Autodesk Fusion 360 part; units mm, degrees
(part 3 of 3)
sketch "Sketch33" plane through (0, 0, 2.9845) normal (0, 0, 1) x (1, 0, 0)
  line L0 (32.131, 76.2) -> (38.1, 76.2)
  line L1 (38.1, 76.2) -> (38.1, 95.631)
  line L2 (38.1, 95.631) -> (32.131, 95.631)
  line L3 (32.131, 95.631) -> (32.131, 101.6)
  line L4 (32.131, 101.6) -> (38.1, 101.6)
  line L5 (38.1, 101.6) -> (38.1, 121.031)
  line L6 (38.1, 121.031) -> (32.131, 121.031)
  line L7 (32.131, 121.031) -> (32.131, 127)
  line L8 (32.131, 127) -> (38.1, 127)
  line L9 (38.1, 127) -> (38.1, 146.431)
  line L10 (38.1, 146.431) -> (32.131, 146.431)
  line L11 (32.131, 146.431) -> (32.131, 152.4)
  line L12 (32.131, 152.4) -> (38.1, 152.4)
  line L13 (38.1, 152.4) -> (38.1, 171.831)
  line L14 (38.1, 171.831) -> (32.131, 171.831)
  line L15 (32.131, 171.831) -> (32.131, 177.8)
  line L16 (32.131, 177.8) -> (38.1, 177.8)
  line L17 (38.1, 177.8) -> (38.1, 197.231)
  line L18 (38.1, 197.231) -> (32.131, 197.231)
  line L19 (32.131, 197.231) -> (32.131, 203.2)
  line L20 (32.131, 203.2) -> (38.1, 203.2)
  line L21 (38.1, 203.2) -> (38.1, 222.631)
  line L22 (38.1, 222.631) -> (32.131, 222.631)
  line L23 (32.131, 222.631) -> (32.131, 228.6)
  line L24 (32.131, 228.6) -> (38.1, 228.6)
  line L25 (38.1, 228.6) -> (38.1, 254)
  line L26 (38.1, 254) -> (31.75, 254)
  line L27 (31.75, 254) -> (31.75, 292.1)
  arc A0 (31.75, 292.1) -> (19.05, 304.8) centre (19.05, 292.1) ccw
  line L28 (19.05, 304.8) -> (-19.05, 304.8)
  arc A1 (-19.05, 304.8) -> (-31.75, 292.1) centre (-19.05, 292.1) ccw
  line L29 (-31.75, 292.1) -> (-31.75, 254)
  line L30 (-31.75, 254) -> (-38.1, 254)
  line L31 (-38.1, 254) -> (-38.1, 228.6)
  line L32 (-38.1, 228.6) -> (-32.131, 228.6)
  line L33 (-32.131, 228.6) -> (-32.131, 222.631)
  line L34 (-32.131, 222.631) -> (-38.1, 222.631)
  line L35 (-38.1, 222.631) -> (-38.1, 203.2)
  line L36 (-38.1, 203.2) -> (-32.131, 203.2)
  line L37 (-32.131, 203.2) -> (-32.131, 197.231)
  line L38 (-32.131, 197.231) -> (-38.1, 197.231)
  line L39 (-38.1, 197.231) -> (-38.1, 177.8)
  line L40 (-38.1, 177.8) -> (-32.131, 177.8)
  line L41 (-32.131, 177.8) -> (-32.131, 171.831)
  line L42 (-32.131, 171.831) -> (-38.1, 171.831)
  line L43 (-38.1, 171.831) -> (-38.1, 152.4)
  line L44 (-38.1, 152.4) -> (-32.131, 152.4)
  line L45 (-32.131, 152.4) -> (-32.131, 146.431)
  line L46 (-32.131, 146.431) -> (-38.1, 146.431)
  line L47 (-38.1, 146.431) -> (-38.1, 127)
  line L48 (-38.1, 127) -> (-32.131, 127)
  line L49 (-32.131, 127) -> (-32.131, 121.031)
  line L50 (-32.131, 121.031) -> (-38.1, 121.031)
  line L51 (-38.1, 121.031) -> (-38.1, 101.6)
  line L52 (-38.1, 101.6) -> (-32.131, 101.6)
  line L53 (-32.131, 101.6) -> (-32.131, 95.631)
  line L54 (-32.131, 95.631) -> (-38.1, 95.631)
  line L55 (-38.1, 95.631) -> (-38.1, 76.2)
  line L56 (-38.1, 76.2) -> (-32.131, 76.2)
  line L57 (-32.131, 76.2) -> (-32.131, 70.231)
  line L58 (-32.131, 70.231) -> (-38.1, 70.231)
  line L59 (-38.1, 70.231) -> (-38.1, 50.8)
  line L60 (-38.1, 50.8) -> (-32.131, 50.8)
  line L61 (-32.131, 50.8) -> (-32.131, 44.831)
  line L62 (-32.131, 44.831) -> (-38.1, 44.831)
  line L63 (-38.1, 44.831) -> (-38.1, 0)
  line L64 (-38.1, 0) -> (-88.9, 0)
  line L65 (-88.9, 0) -> (-88.9, 5.969)
  line L66 (-88.9, 5.969) -> (-114.3, 5.969)
  line L67 (-114.3, 5.969) -> (-114.3, -6.35)
  arc A2 (-114.3, -6.35) -> (-101.6, -19.05) centre (-101.6, -6.35) ccw
  line L68 (-101.6, -19.05) -> (-2.9845, -19.05)
  line L69 (-2.9845, -19.05) -> (-2.9845, -9.525)
  line L70 (-2.9845, -9.525) -> (2.9845, -9.525)
  line L71 (2.9845, -9.525) -> (2.9845, -19.05)
  line L72 (2.9845, -19.05) -> (101.6, -19.05)
  arc A3 (101.6, -19.05) -> (114.3, -6.35) centre (101.6, -6.35) ccw
  line L73 (114.3, -6.35) -> (114.3, 5.969)
  line L74 (114.3, 5.969) -> (88.9, 5.969)
  line L75 (88.9, 5.969) -> (88.9, 0)
  line L76 (88.9, 0) -> (38.1, 0)
  line L77 (38.1, 0) -> (38.1, 44.831)
  line L78 (38.1, 44.831) -> (32.131, 44.831)
  line L79 (32.131, 44.831) -> (32.131, 50.8)
  line L80 (32.131, 50.8) -> (38.1, 50.8)
  line L81 (38.1, 50.8) -> (38.1, 70.231)
  line L82 (38.1, 70.231) -> (32.131, 70.231)
  line L83 (32.131, 70.231) -> (32.131, 76.2)
  circle A4 centre (17.3609, 285.75) radius 11.1125
  circle A5 centre (-17.3609, 285.75) radius 11.1125
sketch "Sketch34" plane through (2.9845, 0, 0) normal (1, 0, 0) x (0, 0, -1)
  circle A0 centre (-17.3736, 285.75) radius 11.1125
  circle A1 centre (17.3736, 285.75) radius 11.1125
  line L0 (-38.1, 76.2) -> (-32.131, 76.2)
  line L1 (-32.131, 76.2) -> (-32.131, 70.231)
  line L2 (-32.131, 70.231) -> (-38.1, 70.231)
  line L3 (-38.1, 70.231) -> (-38.1, 50.8)
  line L4 (-38.1, 50.8) -> (-32.131, 50.8)
  line L5 (-32.131, 50.8) -> (-32.131, 44.831)
  line L6 (-32.131, 44.831) -> (-38.1, 44.831)
  line L7 (-38.1, 44.831) -> (-38.1, 0)
  line L8 (-38.1, 0) -> (-88.9, 0)
  line L9 (-88.9, 0) -> (-88.9, 5.969)
  line L10 (-88.9, 5.969) -> (-114.3, 5.969)
  line L11 (-114.3, 5.969) -> (-114.3, -6.35)
  arc A2 (-114.3, -6.35) -> (-101.6, -19.05) centre (-101.6, -6.35) ccw
  line L12 (-101.6, -19.05) -> (101.6, -19.05)
  arc A3 (101.6, -19.05) -> (114.3, -6.35) centre (101.6, -6.35) ccw
  line L13 (114.3, -6.35) -> (114.3, 5.969)
  line L14 (114.3, 5.969) -> (88.9, 5.969)
  line L15 (88.9, 5.969) -> (88.9, 0)
  line L16 (88.9, 0) -> (38.1, 0)
  line L17 (38.1, 0) -> (38.1, 44.831)
  line L18 (38.1, 44.831) -> (32.131, 44.831)
  line L19 (32.131, 44.831) -> (32.131, 50.8)
  line L20 (32.131, 50.8) -> (38.1, 50.8)
  line L21 (38.1, 50.8) -> (38.1, 70.231)
  line L22 (38.1, 70.231) -> (32.131, 70.231)
  line L23 (32.131, 70.231) -> (32.131, 76.2)
  line L24 (32.131, 76.2) -> (38.1, 76.2)
  line L25 (38.1, 76.2) -> (38.1, 95.631)
  line L26 (38.1, 95.631) -> (32.131, 95.631)
  line L27 (32.131, 95.631) -> (32.131, 101.6)
  line L28 (32.131, 101.6) -> (38.1, 101.6)
  line L29 (38.1, 101.6) -> (38.1, 121.031)
  line L30 (38.1, 121.031) -> (32.131, 121.031)
  line L31 (32.131, 121.031) -> (32.131, 127)
  line L32 (32.131, 127) -> (38.1, 127)
  line L33 (38.1, 127) -> (38.1, 146.431)
  line L34 (38.1, 146.431) -> (32.131, 146.431)
  line L35 (32.131, 146.431) -> (32.131, 152.4)
  line L36 (32.131, 152.4) -> (38.1, 152.4)
  line L37 (38.1, 152.4) -> (38.1, 171.831)
  line L38 (38.1, 171.831) -> (32.131, 171.831)
  line L39 (32.131, 171.831) -> (32.131, 177.8)
  line L40 (32.131, 177.8) -> (38.1, 177.8)
  line L41 (38.1, 177.8) -> (38.1, 197.231)
  line L42 (38.1, 197.231) -> (32.131, 197.231)
  line L43 (32.131, 197.231) -> (32.131, 203.2)
  line L44 (32.131, 203.2) -> (38.1, 203.2)
  line L45 (38.1, 203.2) -> (38.1, 222.631)
  line L46 (38.1, 222.631) -> (32.131, 222.631)
  line L47 (32.131, 222.631) -> (32.131, 228.6)
  line L48 (32.131, 228.6) -> (38.1, 228.6)
  line L49 (38.1, 228.6) -> (38.1, 254)
  line L50 (38.1, 254) -> (31.75, 254)
  line L51 (31.75, 254) -> (31.75, 292.1)
  arc A4 (31.75, 292.1) -> (19.05, 304.8) centre (19.05, 292.1) ccw
  line L52 (19.05, 304.8) -> (2.9845, 304.8)
  line L53 (2.9845, 304.8) -> (2.9845, -9.525)
  line L54 (2.9845, -9.525) -> (-2.9845, -9.525)
  line L55 (-2.9845, -9.525) -> (-2.9845, 304.8)
  line L56 (-2.9845, 304.8) -> (-19.05, 304.8)
  arc A5 (-19.05, 304.8) -> (-31.75, 292.1) centre (-19.05, 292.1) ccw
  line L57 (-31.75, 292.1) -> (-31.75, 254)
  line L58 (-31.75, 254) -> (-38.1, 254)
  line L59 (-38.1, 254) -> (-38.1, 228.6)
  line L60 (-38.1, 228.6) -> (-32.131, 228.6)
  line L61 (-32.131, 228.6) -> (-32.131, 222.631)
  line L62 (-32.131, 222.631) -> (-38.1, 222.631)
  line L63 (-38.1, 222.631) -> (-38.1, 203.2)
  line L64 (-38.1, 203.2) -> (-32.131, 203.2)
  line L65 (-32.131, 203.2) -> (-32.131, 197.231)
  line L66 (-32.131, 197.231) -> (-38.1, 197.231)
  line L67 (-38.1, 197.231) -> (-38.1, 177.8)
  line L68 (-38.1, 177.8) -> (-32.131, 177.8)
  line L69 (-32.131, 177.8) -> (-32.131, 171.831)
  line L70 (-32.131, 171.831) -> (-38.1, 171.831)
  line L71 (-38.1, 171.831) -> (-38.1, 152.4)
  line L72 (-38.1, 152.4) -> (-32.131, 152.4)
  line L73 (-32.131, 152.4) -> (-32.131, 146.431)
  line L74 (-32.131, 146.431) -> (-38.1, 146.431)
  line L75 (-38.1, 146.431) -> (-38.1, 127)
  line L76 (-38.1, 127) -> (-32.131, 127)
  line L77 (-32.131, 127) -> (-32.131, 121.031)
  line L78 (-32.131, 121.031) -> (-38.1, 121.031)
  line L79 (-38.1, 121.031) -> (-38.1, 101.6)
  line L80 (-38.1, 101.6) -> (-32.131, 101.6)
  line L81 (-32.131, 101.6) -> (-32.131, 95.631)
  line L82 (-32.131, 95.631) -> (-38.1, 95.631)
  line L83 (-38.1, 95.631) -> (-38.1, 76.2)
move_face "OffsetFaces2" offset -152.4 1 faces at (-0.9948, -9.525, 0.9948) on bodies 3 in component "Component'"
sketch "Sketch35" plane through (2.9845, 0, 0) normal (1, 0, 0) x (0, 0, -1)
  circle A0 centre (-17.3736, 285.75) radius 11.1125
  circle A1 centre (17.3736, 285.75) radius 11.1125
  line L0 (-38.1, 76.2) -> (-32.131, 76.2)
  line L1 (-32.131, 76.2) -> (-32.131, 70.231)
  line L2 (-32.131, 70.231) -> (-38.1, 70.231)
  line L3 (-38.1, 70.231) -> (-38.1, 50.8)
  line L4 (-38.1, 50.8) -> (-32.131, 50.8)
  line L5 (-32.131, 50.8) -> (-32.131, 44.831)
  line L6 (-32.131, 44.831) -> (-38.1, 44.831)
  line L7 (-38.1, 44.831) -> (-38.1, 0)
  line L8 (-38.1, 0) -> (-88.9, 0)
  line L9 (-88.9, 0) -> (-88.9, 5.969)
  line L10 (-88.9, 5.969) -> (-114.3, 5.969)
  line L11 (-114.3, 5.969) -> (-114.3, -6.35)
  arc A2 (-114.3, -6.35) -> (-101.6, -19.05) centre (-101.6, -6.35) ccw
  line L12 (-101.6, -19.05) -> (101.6, -19.05)
  arc A3 (101.6, -19.05) -> (114.3, -6.35) centre (101.6, -6.35) ccw
  line L13 (114.3, -6.35) -> (114.3, 5.969)
  line L14 (114.3, 5.969) -> (88.9, 5.969)
  line L15 (88.9, 5.969) -> (88.9, 0)
  line L16 (88.9, 0) -> (38.1, 0)
  line L17 (38.1, 0) -> (38.1, 44.831)
  line L18 (38.1, 44.831) -> (32.131, 44.831)
  line L19 (32.131, 44.831) -> (32.131, 50.8)
  line L20 (32.131, 50.8) -> (38.1, 50.8)
  line L21 (38.1, 50.8) -> (38.1, 70.231)
  line L22 (38.1, 70.231) -> (32.131, 70.231)
  line L23 (32.131, 70.231) -> (32.131, 76.2)
  line L24 (32.131, 76.2) -> (38.1, 76.2)
  line L25 (38.1, 76.2) -> (38.1, 95.631)
  line L26 (38.1, 95.631) -> (32.131, 95.631)
  line L27 (32.131, 95.631) -> (32.131, 101.6)
  line L28 (32.131, 101.6) -> (38.1, 101.6)
  line L29 (38.1, 101.6) -> (38.1, 121.031)
  line L30 (38.1, 121.031) -> (32.131, 121.031)
  line L31 (32.131, 121.031) -> (32.131, 127)
  line L32 (32.131, 127) -> (38.1, 127)
  line L33 (38.1, 127) -> (38.1, 146.431)
  line L34 (38.1, 146.431) -> (32.131, 146.431)
  line L35 (32.131, 146.431) -> (32.131, 152.4)
  line L36 (32.131, 152.4) -> (38.1, 152.4)
  line L37 (38.1, 152.4) -> (38.1, 171.831)
  line L38 (38.1, 171.831) -> (32.131, 171.831)
  line L39 (32.131, 171.831) -> (32.131, 177.8)
  line L40 (32.131, 177.8) -> (38.1, 177.8)
  line L41 (38.1, 177.8) -> (38.1, 197.231)
  line L42 (38.1, 197.231) -> (32.131, 197.231)
  line L43 (32.131, 197.231) -> (32.131, 203.2)
  line L44 (32.131, 203.2) -> (38.1, 203.2)
  line L45 (38.1, 203.2) -> (38.1, 222.631)
  line L46 (38.1, 222.631) -> (32.131, 222.631)
  line L47 (32.131, 222.631) -> (32.131, 228.6)
  line L48 (32.131, 228.6) -> (38.1, 228.6)
  line L49 (38.1, 228.6) -> (38.1, 254)
  line L50 (38.1, 254) -> (31.75, 254)
  line L51 (31.75, 254) -> (31.75, 292.1)
  arc A4 (31.75, 292.1) -> (19.05, 304.8) centre (19.05, 292.1) ccw
  line L52 (19.05, 304.8) -> (2.9845, 304.8)
  line L53 (2.9845, 304.8) -> (2.9845, -9.525)
  line L54 (2.9845, -9.525) -> (-2.9845, -9.525)
  line L55 (-2.9845, -9.525) -> (-2.9845, 304.8)
  line L56 (-2.9845, 304.8) -> (-19.05, 304.8)
  arc A5 (-19.05, 304.8) -> (-31.75, 292.1) centre (-19.05, 292.1) ccw
  line L57 (-31.75, 292.1) -> (-31.75, 254)
  line L58 (-31.75, 254) -> (-38.1, 254)
  line L59 (-38.1, 254) -> (-38.1, 228.6)
  line L60 (-38.1, 228.6) -> (-32.131, 228.6)
  line L61 (-32.131, 228.6) -> (-32.131, 222.631)
  line L62 (-32.131, 222.631) -> (-38.1, 222.631)
  line L63 (-38.1, 222.631) -> (-38.1, 203.2)
  line L64 (-38.1, 203.2) -> (-32.131, 203.2)
  line L65 (-32.131, 203.2) -> (-32.131, 197.231)
  line L66 (-32.131, 197.231) -> (-38.1, 197.231)
  line L67 (-38.1, 197.231) -> (-38.1, 177.8)
  line L68 (-38.1, 177.8) -> (-32.131, 177.8)
  line L69 (-32.131, 177.8) -> (-32.131, 171.831)
  line L70 (-32.131, 171.831) -> (-38.1, 171.831)
  line L71 (-38.1, 171.831) -> (-38.1, 152.4)
  line L72 (-38.1, 152.4) -> (-32.131, 152.4)
  line L73 (-32.131, 152.4) -> (-32.131, 146.431)
  line L74 (-32.131, 146.431) -> (-38.1, 146.431)
  line L75 (-38.1, 146.431) -> (-38.1, 127)
  line L76 (-38.1, 127) -> (-32.131, 127)
  line L77 (-32.131, 127) -> (-32.131, 121.031)
  line L78 (-32.131, 121.031) -> (-38.1, 121.031)
  line L79 (-38.1, 121.031) -> (-38.1, 101.6)
  line L80 (-38.1, 101.6) -> (-32.131, 101.6)
  line L81 (-32.131, 101.6) -> (-32.131, 95.631)
  line L82 (-32.131, 95.631) -> (-38.1, 95.631)
  line L83 (-38.1, 95.631) -> (-38.1, 76.2)
  line L84 (-2.9845, 304.8) -> (-2.9845, 142.875) construction
  line L85 (-2.9845, 142.875) -> (2.9845, 142.875)
  line L86 (2.9845, 142.875) -> (2.9845, -9.525)
  line L87 (2.9845, -9.525) -> (-2.9845, -9.525)
  line L88 (-2.9845, -9.525) -> (-2.9845, 142.875)
  dimension "d323" = 161.925
  dimension "d324" = 152.4
  constraint coincident L55.end L56.start
  constraint perpendicular L56 L84
  constraint horizontal L85
  constraint vertical L86
  constraint horizontal L87
  constraint vertical L88
  measures "d323" distance of L55.end L84.end
  measures "d324" distance of L84.end L54.end
extrude "Extrude13" add sketch "Sketch35" against normal blind 5.969 contours L53 L54 L55 L85 L86 L87 L88 bodies 4 in component "Component''"
component "Component" placed x (1, 0, 0) y (0, 1, 0) z (0, 0, 1) at (0, 0, 0)
component "Component'" placed x (1, 0, 0) y (0, 1, 0) z (0, 0, 1) at (0, 0, 0)
component "Component''" placed x (1, 0, 0) y (0, 1, 0) z (0, 0, 1) at (0, 0, 0)
component "Component'''" placed x (1, 0, 0) y (0, 1, 0) z (0, 0, 1) at (0, 0, 0)
equation "d45 = 1.5 in - ( 0.235 / 2 ) * 1 in"
equation "d48 = 1.5 in - ( 0.235 / 2 ) * 1 in"
equation "d72 = ( 1.133 / 2 ) * 1 in"
equation "d74 = ( 1.133 / 2 ) * 1 in"
equation "d84 = ( 1.133 / 2 ) * 1 in"
equation "d85 = ( 1.133 / 2 ) * 1 in"
equation "d115 = ( 0.235 / 2 ) * 1 in"
equation "d116 = ( 0.235 / 2 ) * 1 in"
